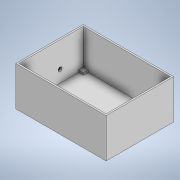
# Autodesk Inventor part: box
Saved by Autodesk Inventor 2021 (Build 250183000, 183)
## iProperties
Created: 2020-11-03
Part Number: box
Material: Generic
Document SubType Name: Modeling
Designer: s094623
Density: 1 g/cm^3
Appearance: Default
Author: s094623
Autodesk Inventor part; units mm, degrees
ref_plane "YZ Plane" through (0, 0, 0) normal (1, 0, 0) x (0, 1, 0)
ref_plane "XZ Plane" through (0, 0, 0) normal (0, 1, 0) x (-1, 0, 0)
ref_plane "XY Plane" through (0, 0, 0) normal (0, 0, 1) x (1, 0, 0)
sketch "Sketch1" plane through (0, 0, 0) normal (0, 1, 0) x (-1, 0, 0)
  line L0 (0, 0) -> (-111, 0)
  line L1 (-111, 0) -> (-111, 82)
  line L2 (-111, 82) -> (0, 82)
  line L3 (0, 82) -> (0, 0)
  dimension "d0" = 111
  dimension "d1" = 82
  constraints: 8 end point, 3 perpendicular, 1 horizontal
  measures "d0" distance of L0.start L0.end
  measures "d1" distance of L0.end L1.end
extrude "Extrusion1" add sketch "Sketch1" along normal blind 2
sketch "Sketch2" plane through (0, 0, 0) normal (0, -1, 0) x (1, 0, 0)
  point P0 (0, 0)
sketch "Sketch3" plane through (0, 0, 0) normal (0, -1, 0) x (1, 0, 0)
  line L0 (0, 0) -> (0, 82) projected
  line L1 (0, 0) -> (0, 82)
  line L2 (0, 82) -> (-2, 82)
  line L3 (-2, 82) -> (-2, 0)
  line L4 (-2, 0) -> (0, 0)
  line L5 (-2, 0) -> (-2, -2)
  line L6 (-2, -2) -> (113, -2)
  line L7 (113, -2) -> (113, 0)
  line L8 (113, 0) -> (-2, 0)
  line L9 (113, 0) -> (113, 84)
  line L10 (113, 84) -> (111, 84)
  line L11 (111, 84) -> (111, -2)
  line L12 (111, 84) -> (-2, 84)
  line L13 (111, 82) -> (111, 0) projected
  line L14 (-2, 82) -> (111, 82)
  line L15 (111, 82) -> (111, 84)
  dimension "d4" = 2
  dimension "d5" = 2
  dimension "d6" = 115
  dimension "d7" = 2
  dimension "d8" = 84
  dimension "d9" = 2
  constraints: 28 end point, 7 perpendicular, 6 point on line, 1 vertical
  measures "d4" distance of L0.end L2.end
  measures "d5" distance of L3.end L5.end
  measures "d6" distance of L5.end L6.end
  measures "d7" distance of L6.end L7.end
  measures "d8" distance of L7.end L9.end
  measures "d9" distance of L9.end L10.end
extrude "Extrusion2" add sketch "Sketch3" against normal blind 50 contours L11 L10 L9 L8
sketch "Sketch4" plane through (0, 0, 0) normal (0, -1, 0) x (1, 0, 0)
  line L0 (111, 84) -> (111, 82) projected
  line L1 (111, 84) -> (-2, 84)
  line L2 (-2, 84) -> (-2, 82)
  line L3 (0, 82) -> (111, 82) projected
  line L4 (-2, 82) -> (111, 82)
  line L5 (111, 82) -> (111, 84)
  point P0 (0, 0)
  dimension "d12" = 113
  constraints: 8 end point, 3 perpendicular, 1 horizontal
  measures "d12" distance of L0.start L1.end
extrude "Extrusion3" add sketch "Sketch4" against normal blind 50
sketch "Sketch5" plane through (0, 0, 0) normal (0, -1, 0) x (1, 0, 0)
  line L0 (-2, 84) -> (-2, 82) projected
  line L1 (-2, 82) -> (-2, -2)
  line L2 (-2, -2) -> (0, -2)
  line L3 (0, 0) -> (0, 82) projected
  line L4 (0, -2) -> (0, 82)
  line L5 (-2, 82) -> (0, 82) projected
  line L6 (0, 82) -> (-2, 82)
  dimension "d15" = 84
  constraints: 8 end point, 2 collinear, 2 perpendicular
  measures "d15" distance of L0.end L1.end
extrude "Extrusion4" add sketch "Sketch5" against normal blind 50
sketch "Sketch6" plane through (0, 0, 0) normal (0, -1, 0) x (1, 0, 0)
  line L0 (0, 0) -> (113, 0) projected
  line L1 (113, 0) -> (113, -2)
  line L2 (0, 82) -> (0, -2) projected
  line L3 (113, -2) -> (0, -2)
  line L4 (0, -2) -> (0, 0)
  dimension "d18" = 2
  constraints: 6 end point, 1 collinear, 1 vertical
  measures "d18" distance of L0.end L1.end
extrude "Extrusion5" add sketch "Sketch6" against normal blind 50
sketch "Sketch7" plane through (-2, 0, 84) normal (-1, 0, 0) x (0, 0, 1)
  circle A0 centre (-54.3, 17.5) radius 2.5
  point P0 (-84, 0)
  dimension "d21" = 5
  constraints: 1 centre point
  measures "d21" diameter of A0
hole "Hole1" at (-2, 17.5, 29.7) direction (1, 0, 0) diameter 5 depth 2 tip angle 118
sketch "Sketch8" plane through (-2, 0, 84) normal (-1, 0, 0) x (0, 0, 1)
  line L0 (-61.8, 10) -> (-61.8, 25)
  line L1 (-61.8, 25) -> (-46.8, 25)
  line L2 (-46.8, 25) -> (-46.8, 10)
  line L3 (-46.8, 10) -> (-61.8, 10)
  point P0 (-84, 0)
  dimension "d29" = 15
  dimension "d30" = 15
  dimension "d31" = 15
  constraints: 8 end point, 2 perpendicular, 1 vertical
  measures "d29" distance of L0.start L0.end
  measures "d30" distance of L0.end L1.end
  measures "d31" distance of L1.end L2.end
extrude "Extrusion6" add sketch "Sketch8" along normal blind 12
chamfer "Chamfer1" distance 10 angle 45 1 edges at (-14, 25, 29.7)
sketch "Sketch9" plane through (-2, 10, 22.2) normal (0, -1, 0) x (1, 0, 0)
  line L0 (0, 0) -> (0, 15) projected
  line L1 (0, 2) -> (-10, 2)
  line L2 (-12, 0) -> (-12, 15) projected
  line L3 (-10, 2) -> (-10, 13)
  line L4 (0, 15) -> (-12, 15) projected
  line L5 (-10, 13) -> (0, 13)
  line L6 (0, 13) -> (0, 2)
  point P0 (2, -22.2)
  point P1 (0, 13)
  dimension "d37" = 10
  dimension "d38" = 11
  constraints: 8 end point, 4 perpendicular, 1 point on line
  measures "d37" distance of L1.start L1.end
  measures "d38" distance of L1.end L3.end
extrude "Extrusion7" cut sketch "Sketch9" against normal blind 13
sketch "Sketch10" plane through (-14, 15, 22.2) normal (-0.7071, 0.7071, 0) x (-0.7071, -0.7071, 0)
  line L0 (-14.1421, 15) -> (-14.1421, 0) projected
  line L1 (-14.1421, 0) -> (-14.1421, 15)
  line L2 (0, 0) -> (0, 15) projected
  line L3 (-14.1421, 15) -> (0, 15)
  line L4 (0, 15) -> (0, 0)
  line L5 (-14.1421, 0) -> (0, 0) projected
  line L6 (0, 0) -> (-14.1421, 0)
  point P0 (0.7071, -22.2)
  constraints: 8 end point, 2 perpendicular, 1 collinear, 1 vertical
extrude "Extrusion8" add sketch "Sketch10" along normal blind 2
chamfer "Chamfer2" distance 2 angle 45 1 edges at (-5.4142, 26.4142, 29.7)
chamfer "Chamfer3" distance 2 angle 45 1 edges at (-15.4142, 16.4142, 29.7)
sketch "Sketch11" plane through (0, 2, 0) normal (0, 1, 0) x (1, 0, 0)
  line L0 (0, 0) -> (0, -82) projected
  line L1 (0, 0) -> (0, -6)
  line L2 (0, -6) -> (6, -6)
  line L3 (6, -6) -> (6, 0)
  line L4 (0, 0) -> (111, 0) projected
  line L5 (6, 0) -> (0, 0)
  dimension "d49" = 6
  dimension "d50" = 6
  dimension "d51" = 6
  constraints: 8 end point, 2 point on line, 1 collinear, 1 perpendicular
  measures "d49" distance of L0.start L1.end
  measures "d50" distance of L1.end L2.end
  measures "d51" distance of L2.end L3.end
extrude "Extrusion9" add sketch "Sketch11" along normal blind 3
sketch "Sketch12" plane through (0, 2, 0) normal (0, 1, 0) x (1, 0, 0)
  point P0 (0, 0)
sketch "Sketch13" plane through (0, 2, 0) normal (0, 1, 0) x (1, 0, 0)
  line L0 (111, 0) -> (111, -6)
  line L1 (111, 0) -> (111, -82) projected
  line L2 (111, -6) -> (105, -6)
  line L3 (105, -6) -> (105, 0)
  line L4 (0, 0) -> (111, 0) projected
  line L5 (105, 0) -> (111, 0)
  dimension "d54" = 6
  dimension "d55" = 6
  constraints: 8 end point, 2 perpendicular, 1 collinear, 1 point on line
  measures "d54" distance of L0.start L0.end
  measures "d55" distance of L0.end L2.end
extrude "Extrusion10" add sketch "Sketch13" along normal blind 3
sketch "Sketch14" plane through (0, 2, 0) normal (0, 1, 0) x (1, 0, 0)
  point P0 (0, 0)
sketch "Sketch15" plane through (0, 2, 0) normal (0, 1, 0) x (1, 0, 0)
  line L0 (0, -82) -> (111, -82) projected
  line L1 (0, -82) -> (0, -76)
  line L2 (0, -6) -> (0, -82) projected
  line L3 (0, -76) -> (6, -76)
  line L4 (6, -76) -> (6, -82)
  point P0 (0, 0)
  dimension "d58" = 6
  dimension "d59" = 6
  constraints: 6 end point, 2 point on line, 1 horizontal, 1 perpendicular
  measures "d58" distance of L0.start L1.end
  measures "d59" distance of L1.end L3.end
extrude "Extrusion11" add sketch "Sketch15" along normal blind 3
sketch "Sketch16" plane through (0, 2, 0) normal (0, 1, 0) x (1, 0, 0)
  line L0 (111, -82) -> (0, -82) projected
  line L1 (111, -82) -> (111, -76)
  line L2 (111, 0) -> (111, -82) projected
  line L3 (111, -76) -> (105, -76)
  line L4 (105, -76) -> (105, -82)
  line L5 (105, -82) -> (111, -82)
  point P0 (0, 0)
  dimension "d62" = 6
  dimension "d63" = 6
  constraints: 8 end point, 3 perpendicular, 1 point on line
  measures "d62" distance of L0.start L1.end
  measures "d63" distance of L1.end L3.end
extrude "Extrusion12" add sketch "Sketch16" along normal blind 3
body "Solid1"
